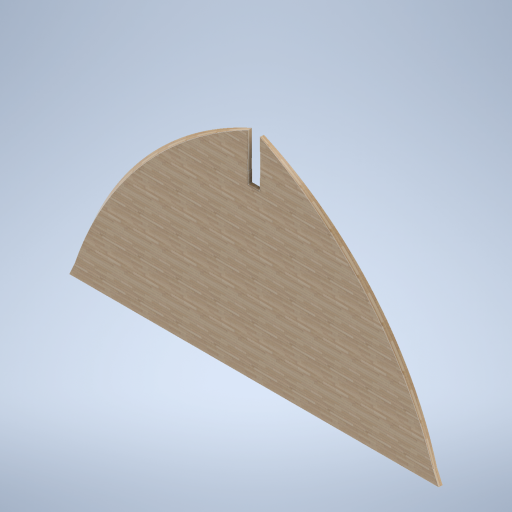
# Autodesk Inventor part: curve_front_wall
Saved by Autodesk Inventor 2024.2 (Build 282272000, 272)
## iProperties
Created: 2024-05-21
Part Number: curve_front_wall
Material: Wood (Maple)
Document SubType Name: Modeling
Designer: LOSTER_1
Density: 0.67 g/cm^3
Appearance: Natural Maple - Glossy Dark Tint
Author: LOSTER_1
Autodesk Inventor part; units mm, degrees
ref_plane "YZ Plane" through (0, 0, 0) normal (1, 0, 0) x (0, 1, 0)
ref_plane "XZ Plane" through (0, 0, 0) normal (0, 1, 0) x (-1, 0, 0)
sketch "Sketch1" plane through (0, 0, 0) normal (0, 0, 1) x (1, 0, 0)
  ellipse E0 centre (3111.3517, -3183.1732) end of major axis (3111.3517, 4817.0015) minor radius 8000.1746 (-159.7881, 4117.6788) -> (-165.4979, 4115.1179) ccw construction
  arc A0 (-159.7998, 4117.6867) -> (-4592.5379, -1035.3503) centre (3941.5776, -3893.4745) ccw
  ellipse E1 centre (3109.6714, -4630.6209) end of major axis (3109.6714, 3869.3791) minor radius 8499.9999 (-4592.5379, -1035.3503) -> (-4736.8993, -1362.3911) ccw
  line L0 (-159.7998, 4117.6867) -> (-166.4305, 3212.6664)
  arc A1 (4572.962, -1035.3503) -> (140.224, 4117.6867) centre (-3961.1534, -3893.4745) ccw
  ellipse E2 centre (-3129.2472, -4630.6209) end of major axis (-3129.2472, 3869.3791) minor radius 8499.9999 (4717.3235, -1362.3911) -> (4572.962, -1035.3503) ccw
  line L1 (140.224, 4117.6867) -> (146.8547, 3212.6664)
  line L2 (-4736.8993, -1362.3911) -> (4717.3235, -1362.3911)
  line L3 (-159.7879, 3212.6664) -> (-159.7879, 2912.6664)
  line L4 (-159.7879, 2912.6664) -> (140.2121, 2912.6664)
  line L5 (140.2121, 2912.6664) -> (140.2121, 3212.6664)
  line L6 (-166.4305, 3212.6664) -> (-159.7879, 3212.6664)
  line L7 (140.2121, 3212.6664) -> (146.8547, 3212.6664)
  point P0 (0, 0)
  point P1 (-9.7879, 2912.6664)
  constraints: 16 end point, 4 point on circle, 3 perpendicular, 2 centre point, 1 collinear, 1 horizontal, 1 vertical, 14 other
ref_plane "Work Plane2" through (0, 0, -100) normal (0, 0, 1) x (1, 0, 0)
ref_plane "Work Plane1" through (0, 0, 0) normal (0, 0, 1) x (1, 0, 0)
sketch "Sketch3" plane through (0, 0, -100) normal (0, 0, 1) x (1, 0, 0)
  ellipse E0 centre (3111.3517, -3183.1732) end of major axis (3111.3517, 4817.0015) minor radius 8000.1746 (-165.4979, 4115.1179) -> (-1490.8772, 3360.7006) ccw construction
  line L0 (-159.7879, 2912.6664) -> (-9.7879, 2912.6664)
  line L1 (-159.7879, 3212.6664) -> (-159.7879, 2912.6664)
  ellipse E1 centre (-3129.2472, -4630.6209) end of major axis (-3129.2472, 3869.3791) minor radius 8499.9999 (4717.3235, -1362.3911) -> (4572.962, -1035.3503) ccw projected
  ellipse E2 centre (3109.6714, -4630.6209) end of major axis (3109.6714, 3869.3791) minor radius 8499.9999 (-4592.5379, -1035.3503) -> (-4736.8993, -1362.3911) ccw projected
  arc A0 (-4592.5379, -1035.3503) -> (-4736.8993, -1362.3911) centre (3109.6716, -4630.6209) ccw
  arc A1 (-165.4979, 4115.1179) -> (-4592.5379, -1035.3503) centre (3108.2023, -3176.6084) ccw
  line L2 (140.2121, 3212.6664) -> (140.2121, 2912.6664)
  line L3 (145.9221, 4115.1179) -> (146.8547, 3212.6664)
  arc A2 (4717.3235, -1362.3911) -> (4572.962, -1035.3503) centre (-3129.2474, -4630.6209) ccw
  arc A3 (4572.962, -1035.3503) -> (145.9221, 4115.1179) centre (-3127.7781, -3176.6084) ccw
  line L4 (-9.7879, 2912.6664) -> (140.2121, 2912.6664)
  line L5 (-4736.8993, -1362.3911) -> (4717.3235, -1362.3911)
  line L6 (-159.7879, 3212.6664) -> (-166.7879, 3212.6664)
  line L7 (-166.7879, 3212.6664) -> (-165.4979, 4115.1179)
  line L8 (146.8547, 3212.6664) -> (140.2121, 3212.6664)
  point P0 (0, 0)
  point P1 (-9.7879, 3107.3885)
  dimension "d5" = 7
  constraints: 18 end point, 8 point on circle, 7 coincident, 4 centre point, 4 horizontal, 3 other
  measures "d5" distance of L1.start L6.end
loft "Loft1" add profiles "Sketch3", "Sketch1"
body "Solid1"
